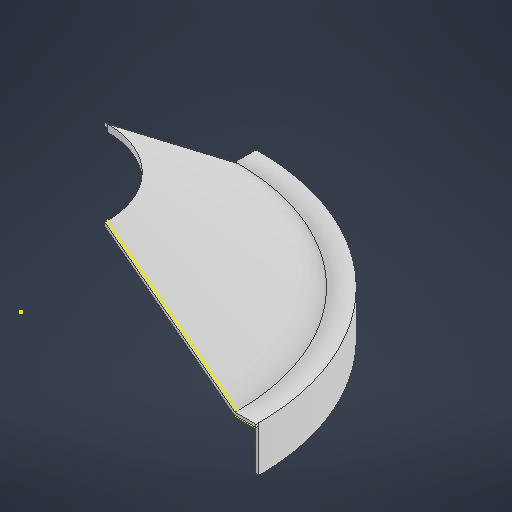
# Autodesk Inventor part: Cover_v1
Saved by Autodesk Inventor 2026.2 (Build 302298000, 298)
## iProperties
Created: 2025-12-11
Part Number: Cover_v1
Material: Generic
Document SubType Name: Modeling
Designer: Thoma
Density: 1 g/cm^3
Appearance: Default
Author: Thoma
Autodesk Inventor part; units mm, degrees
ref_plane "YZ Plane" through (0, 0, 0) normal (1, 0, 0) x (0, 1, 0)
ref_plane "XZ Plane" through (0, 0, 0) normal (0, 1, 0) x (-1, 0, 0)
ref_plane "XY Plane" through (0, 0, 0) normal (0, 0, 1) x (1, 0, 0)
sketch "Sketch1" plane through (0, 0, 0) normal (1, 0, 0) x (0, 1, 0)
  line L0 (0, 0) -> (0, -104)
  line L1 (79.3684, 0) -> (0, -104)
  line L2 (79.3684, 0) -> (0, 0)
  line L3 (0, -104) -> (0, -104)
  line L4 (0, -104) -> (0, -106)
  line L5 (0, -106) -> (0, -106)
  line L6 (12, -88.2759) -> (12, -121.4374)
  line L7 (17, -106) -> (0, -106)
  line L8 (17, -104) -> (0, -104)
  line L9 (85.6581, 0) -> (17, -89.9658)
  line L10 (105.5294, 0) -> (79.3684, 0)
  line L11 (17, -89.9658) -> (17, -119.3457)
  circle A0 centre (12, -106) radius 2
  point P0 (12, -104)
  point P1 (14, -106)
  dimension "d5" = 79.3684
  dimension "d6" = 104
  dimension "d7" = 12
  dimension "d8" = 88.2759
  dimension "d9" = 0
  dimension "d11" = 2
  dimension "d12" = 5
  dimension "d13" = 5
  constraints: 24 end point, 9 point on line, 4 vertical, 2 horizontal, 2 perpendicular, 1 centre point, 1 collinear, 1 parallel
  measures "d5" distance of L0.start L1.start
  measures "d6" distance of L0.start L0.end
  measures "d7" distance from line of L0 L6.start
  measures "d8" distance from line of L6.start L2
  measures "d9" distance from line of L0 L3.start
  measures "d11" distance of L3.start L4.end
  measures "d12" distance between parallel lines of L9 L1
  measures "d13" distance between parallel lines of L6 L11
extrude "Extrusion1" add sketch "Sketch1" along normal blind 2 contours L10 L9 L11 L8 L6 L1 | L8 L11 L7 A0
sketch "Sketch2" plane through (2, 0, 0) normal (1, 0, 0) x (0, 0, -1)
  line L0 (0, 85.6581) -> (0, 79.3684) projected
  line L1 (0, 80.6581) -> (89.9658, 12)
  line L2 (88.2759, 12) -> (104, 12) projected
  line L3 (0, 79.3684) -> (88.2759, 12) projected
  line L4 (102.4983, 12) -> (102.4983, 15.9748)
  line L5 (89.9658, 17) -> (0, 85.6581) projected
  line L6 (106, 14) -> (106, 17) projected
  line L7 (106, 15.9748) -> (91.3092, 15.9748)
  line L8 (0, 85.6581) -> (91.3092, 15.9748)
  line L9 (106, 15.9748) -> (106, 17)
  line L10 (106, 17) -> (89.9658, 17) projected
  line L11 (106, 15.9748) -> (106, 17)
  line L12 (106, 17) -> (89.9658, 17)
  point P0 (0, 0)
  dimension "d18" = 5
  dimension "d19" = 3.9748
  dimension "d20" = 3.9748
  constraints: 14 end point, 4 point on line, 2 vertical, 1 collinear, 1 horizontal, 1 parallel, 1 perpendicular
  measures "d18" distance of L1.start L0.start
  measures "d19" distance of L4.start L4.end
  measures "d20" distance between parallel lines of L1 L5
extrude "Extrusion2" cut sketch "Sketch2" against normal blind 2 contours L1 L2 L3 L0 | L10 L6 L7 L8
sketch "Sketch3" plane through (2, 0, 0) normal (1, 0, 0) x (0, 0, -1)
  line L0 (91.3092, 15.9748) -> (0, 85.6581) projected
  line L1 (0, 85.6581) -> (91.3092, 15.9748)
  line L2 (91.3092, 15.9748) -> (106, 15.9748) projected
  line L3 (91.3092, 15.9748) -> (106, 15.9748)
  arc A0 (106, 14) -> (104, 12) centre (106, 12) ccw projected
  line L4 (106, 15.9748) -> (106, 14)
  circle A1 centre (106, 12) radius 2
  line L5 (89.9658, 12) -> (104, 12) projected
  line L6 (89.9658, 12) -> (104, 12)
  line L7 (0, 85.6581) -> (0, 80.6581) projected
  line L8 (0, 85.6581) -> (0, 80.6581)
  line L9 (0, 80.6581) -> (89.9658, 12)
  line L10 (0, 83.1581) -> (-58.5, 83.1581)
  line L11 (0, 85.6581) -> (0, 80.6581) projected
  line L12 (-58.5, 83.1581) -> (-58.5, 115.0333)
  line L13 (106, 14) -> (104, 14)
  line L14 (104, 14) -> (104, -16)
  line L15 (104, -16) -> (106, -16)
  line L16 (106, -16) -> (106, 14)
  line L17 (89.9658, 12) -> (89.9658, 145)
  line L18 (0, 83.1581) -> (89.9658, 83.1581)
  point P0 (0, 0)
  dimension "d21" = 58.5
  dimension "d32" = 30
  dimension "d42" = 89.9658
  constraints: 28 end point, 4 collinear, 4 perpendicular, 3 parallel, 2 horizontal, 2 point on line, 2 vertical, 1 centre point, 1 coincident, 1 concentric, 1 midpoint
  measures "d21" distance of L10.start L10.end
  measures "d32" distance of L15.end L4.end
  measures "d42" distance of L10.start L18.end
revolve "Revolution1" add sketch "Sketch3" angle 90 about axis through (2, 83.1581, 58.5) along (0, -1, 0) contours L2 L4 L13 L14 L5 L17 L0 | L17 L9 L7 L18 L0 | L18 L7 L0 | L16 A1 A0 | A0 L14 L13 | A1 L16 L15 L14
sketch "Sketch14" plane through (166.5, -16, 58.5) normal (0, 0, 1) x (1, 0, 0)
  line L0 (-14.6908, 31.9748) -> (-106, 101.6581) projected
  line L1 (-106, 96.6581) -> (-16.0342, 28) projected
  line L2 (-106, 101.6581) -> (-106, 96.6581)
  line L3 (-16.0342, 28) -> (-2, 28) projected
  line L4 (-106, 96.6581) -> (-16.0342, 28)
  point P0 (-166.5, 16)
  constraints: 4 end point, 1 vertical
sketch "Sketch4" plane through (60.5, 80.6581, 58.5) normal (0, 0, 1) x (1, 0, 0)
  line L0 (0, 5) -> (0, 0) projected
  line L1 (0, 5) -> (0, 0)
  line L2 (0, 0) -> (89.9658, -68.6581) projected
  line L3 (0, 0) -> (89.9658, -68.6581)
  line L4 (89.9658, -68.6581) -> (104, -68.6581) projected
  line L5 (89.9658, -68.6581) -> (104, -68.6581)
  line L6 (106, -66.6581) -> (106, -64.6834) projected
  line L7 (106, -66.6581) -> (106, -64.6834)
  line L8 (91.3092, -64.6834) -> (0, 5) projected
  line L9 (106, -64.6834) -> (91.3092, -64.6834)
  line L10 (91.3092, -64.6834) -> (0, 5)
  arc A0 (106, -66.6581) -> (104, -68.6581) centre (106, -68.6581) ccw projected
  circle A1 centre (106, -68.6581) radius 2
  point P0 (-60.5, -80.6581)
  constraints: 12 end point, 5 collinear, 1 centre point, 1 coincident, 1 perpendicular
extrude "Extrusion3" add sketch "Sketch4" along normal blind 2 contours L8 L9 L6 A0 L4 L2 L0
sketch "Sketch5" plane through (60.5, 80.6581, 60.5) normal (0, 0, 1) x (1, 0, 0)
  line L0 (0, 5) -> (0, 0) projected
  line L1 (0, 2.5) -> (90.621, -66.6581)
  line L2 (-58.5, -66.6581) -> (106, -66.6581) projected
  line L3 (91.3092, -64.6834) -> (0, 5) projected
  line L4 (90.621, -66.6581) -> (106, -66.6581)
  line L5 (106, -66.6581) -> (106, -64.6834) projected
  line L6 (106, -64.6834) -> (91.3092, -64.6834) projected
  line L7 (106, -64.6834) -> (91.3092, -64.6834)
  line L8 (-58.5, 5) -> (0, 5) projected
  line L9 (91.3092, -64.6834) -> (0, 5)
  line L10 (0, 5) -> (0, 2.5)
  line L11 (0, 0) -> (89.9658, -68.6581) projected
  line L12 (89.9658, -68.6581) -> (106, -68.6581)
  line L13 (89.9658, -68.6581) -> (104, -68.6581) projected
  line L14 (106, -68.6581) -> (106, -66.6581)
  line L15 (90.621, -66.6581) -> (0, 2.5)
  line L16 (0, 0) -> (89.9658, -68.6581)
  point P0 (-60.5, -80.6581)
  constraints: 18 end point, 2 collinear, 2 horizontal, 2 parallel, 2 perpendicular, 1 midpoint, 1 point on line
extrude "Extrusion4" cut sketch "Sketch5" against normal blind 2 contours L1 L2 L11 L0 | L2 L14 L12 L11
sketch "Sketch6" plane through (0, 0, 0) normal (-1, 0, 0) x (0, 0, 1)
  line L0 (0, 85.6581) -> (0, 80.6581) projected
  line L1 (0, 83.1581) -> (-90.621, 14)
  line L2 (-106, 14) -> (58.5, 14) projected
  line L3 (-91.3092, 15.9748) -> (0, 85.6581) projected
  line L4 (-106, 14) -> (-106, 15.9748) projected
  line L5 (-90.621, 14) -> (-106, 14)
  line L6 (-106, 14) -> (-106, 15.9748)
  line L7 (-106, 15.9748) -> (-91.3092, 15.9748)
  line L8 (0, 85.6581) -> (0, 83.1581)
  line L9 (-89.9658, 12) -> (58.5, 12) projected
  line L10 (-89.9658, 12) -> (-106, 12)
  line L11 (-104, 12) -> (58.5, 12) projected
  line L12 (-106, 12) -> (-106, 14)
  line L13 (-90.621, 14) -> (0, 83.1581)
  line L14 (0, 80.6581) -> (-89.9658, 12)
  point P0 (0, 0)
  constraints: 18 end point, 3 collinear, 3 parallel, 3 perpendicular, 1 midpoint, 1 point on line
extrude "Extrusion5" cut sketch "Sketch6" against normal blind 2 contours L0 L14 L2 L1 | L2 L14 L10 L12
equation "\"d19\" = d20"
body "Solid1"
